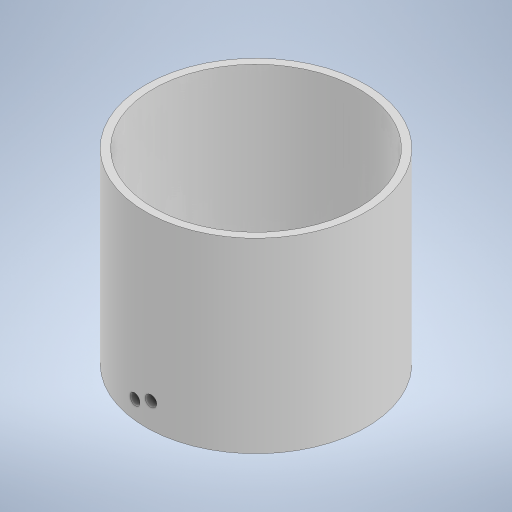
# Autodesk Inventor part: Simple Pressure Gauge Cup 23-02-03
Saved by Autodesk Inventor 2023 (Build 270158000, 158)
## iProperties
Created: 2023-02-03
Part Number: Simple Pressure Gauge Cup 23-02-03
Material: Generic
Document SubType Name: Modeling
Designer: Mikayla
Density: 1 g/cm^3
Appearance: Default
Author: Mikayla
Autodesk Inventor part; units mm, degrees
ref_plane "YZ Plane" through (0, 0, 0) normal (1, 0, 0) x (0, 1, 0)
ref_plane "XZ Plane" through (0, 0, 0) normal (0, 1, 0) x (-1, 0, 0)
sketch "Sketch1" plane through (0, 0, 0) normal (0, 1, 0) x (-1, 0, 0)
  circle A0 centre (0, 0) radius 30
  dimension "d0" = 60
  constraints: 1 centre point, 1 coincident
  measures "d0" diameter of A0
extrude "Extrusion1" add sketch "Sketch1" along normal blind 50.8
shell "Shell1" thickness 2 removed faces 1 at (-9.4188, 50.8, 0)
ref_plane "Work Plane1" through (0, 0, 30) normal (0, 0, 1) x (1, 0, 0)
sketch "Sketch2" plane through (0, 0, 30) normal (0, 0, 1) x (1, 0, 0)
  line L0 (28, 2) -> (-28, 2) projected
  circle A0 centre (-3.1214, 5) radius 1.5
  circle A1 centre (1.3586, 6.9) radius 1.5
  point P0 (0, 0)
  dimension "d4" = 3
  dimension "d5" = 3
  dimension "d6" = 4.48
  dimension "d7" = 1.9
  dimension "d8" = 3
  constraints: 2 centre point
  measures "d4" diameter of A0
  measures "d5" diameter of A1
  measures "d6" horizontal distance of A1.centre A0.centre
  measures "d7" vertical distance of A1.centre A0.centre
  measures "d8" distance from line of L0 A0.centre
extrude "Extrusion2" cut sketch "Sketch2" against normal blind 4
body "Solid1"
